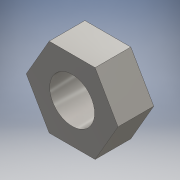
# Autodesk Inventor part: nut3point9mm
Saved by Autodesk Inventor 2016 (Build 200138000, 138)
## iProperties
Created: 2016-06-04
Part Number: nut3point9mm
Material: Stainless Steel
Document SubType Name: Modeling
Designer: hesaon
Density: 8 g/cm^3
Appearance: Semi-Polished
Author: hesaon
Autodesk Inventor part; units mm, degrees
ref_plane "YZ Plane" through (0, 0, 0) normal (1, 0, 0) x (0, 1, 0)
ref_plane "XZ Plane" through (0, 0, 0) normal (0, 1, 0) x (-1, 0, 0)
ref_plane "XY Plane" through (0, 0, 0) normal (0, 0, 1) x (1, 0, 0)
sketch "Sketch1" plane through (0, 0, 0) normal (0, 1, 0) x (-1, 0, 0)
  circle A0 centre (0, 0) radius 1.95
  line L0 (-1.9919, -3.45) -> (-3.9837, 0)
  line L1 (-3.9837, 0) -> (-1.9919, 3.45)
  line L2 (-1.9919, 3.45) -> (1.9919, 3.45)
  line L3 (1.9919, 3.45) -> (3.9837, 0)
  line L4 (3.9837, 0) -> (1.9919, -3.45)
  line L5 (1.9919, -3.45) -> (-1.9919, -3.45)
  dimension "d0" = 3.9
  dimension "d1" = 6.9
  constraints: 12 end point, 2 coincident, 1 centre point, 1 horizontal, 13 other
  measures "d0" diameter of A0
  measures "d1" distance between parallel lines of L2 L5
extrude "Extrusion1" add sketch "Sketch1" along normal blind 3.1
body "Solid1"
